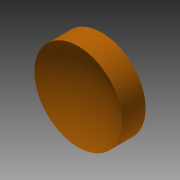
# Autodesk Inventor part: Pip
Saved by Autodesk Inventor 2013 (Build 170138000, 138)
## iProperties
Created: 2013-09-03
Part Number: Pip
Material: Generic
Document SubType Name: Modeling
Designer: s601298
Density: 1 g/cm^3
Author: s601298
Autodesk Inventor part; units mm, degrees
ref_plane "YZ Plane" through (0, 0, 0) normal (1, 0, 0) x (0, 1, 0)
ref_plane "XZ Plane" through (0, 0, 0) normal (0, 1, 0) x (-1, 0, 0)
ref_plane "XY Plane" through (0, 0, 0) normal (0, 0, 1) x (1, 0, 0)
sketch "Sketch1" plane through (0, 0, 0) normal (1, 0, 0) x (0, 1, 0)
  line L0 (-7.9348, -6.3734) -> (-7.9348, -5.7384)
  line L1 (-7.9348, -6.3734) -> (-7.2998, -6.3734) construction
  line L2 (-7.9348, -6.3734) -> (-5.5599, -6.3734)
  line L3 (-5.5599, -5.1034) -> (-5.5599, -6.3734)
  arc A0 (-7.9348, -5.7384) -> (-5.5599, -5.1034) centre (-7.8542, -1.2813) ccw
  point P0 (0, 0)
  dimension "d0" = 0.635
  dimension "d1" = 90
  dimension "d2" = 2.3749
  dimension "d3" = 1.27
  constraints: 8 end point, 2 perpendicular, 2 point on circle, 1 centre point, 1 horizontal, 1 point on line, 1 vertical
  measures "d0" distance of L0.start L0.end
  measures "d1" angle of L1 L0
  measures "d2" distance of L0.start L2.end
  measures "d3" distance of L3.start L2.end
revolve "Revolution1" add sketch "Sketch1" angle 360 about axis through (0, -7.9348, -6.3734) along (0, 0, 1)
body "Solid1"
